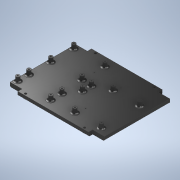
# Autodesk Inventor part: Base_Componentes_Arduino
Saved by Autodesk Inventor 2020 (Build 240168000, 168)
## iProperties
Created: 2021-06-24
Part Number: Base_Componentes_Arduino
Material: Plástico PC/ABS
Document SubType Name: Modeling
Designer: JCarlos
Density: 0.357273 g/cm^3
Appearance: Brilhosa - Preta
Author: JCarlos
Autodesk Inventor part; units mm, degrees
ref_plane "YZ Plane" through (0, 0, 0) normal (1, 0, 0) x (0, 1, 0)
ref_plane "XZ Plane" through (0, 0, 0) normal (0, 1, 0) x (-1, 0, 0)
ref_plane "XY Plane" through (0, 0, 0) normal (0, 0, 1) x (1, 0, 0)
sketch "Esboço1" plane through (0, 0, 0) normal (0, 1, 0) x (-1, 0, 0)
  line L0 (60, -62.5) -> (-60, -62.5)
  line L1 (-80, -55.5) -> (-80, 55.5)
  line L2 (-60, 62.5) -> (60, 62.5)
  line L3 (80, 55.5) -> (80, -55.5)
  line L4 (80, -55.5) -> (60, -55.5)
  line L5 (60, -55.5) -> (60, -62.5)
  line L6 (0, 0) -> (0, -37.6939)
  line L7 (0, 0) -> (28.8208, 0)
  line L8 (-80, -55.5) -> (-60, -55.5)
  line L9 (-60, -55.5) -> (-60, -62.5)
  line L10 (80, 55.5) -> (60, 55.5)
  line L11 (60, 55.5) -> (60, 62.5)
  line L12 (-60, 55.5) -> (-60, 62.5)
  line L13 (-80, 55.5) -> (-60, 55.5)
  point P0 (80, 0)
  point P1 (0, -62.5)
  point P2 (-80, 0)
  point P3 (80, 0)
  dimension "d2" = 7
  dimension "d4" = 20
  dimension "d5" = 125
  dimension "d6" = 111
  dimension "d7" = 160
  constraints: 28 end point, 9 symmetric about line, 4 midpoint, 3 horizontal, 3 horizontal alignment, 2 parallel, 2 perpendicular, 1 point on line, 1 vertical, 1 vertical alignment
  measures "d2" distance between parallel lines of L0 L4
  measures "d4" distance of L3.end L4.end
  measures "d5" distance between parallel lines of L2 L0
  measures "d6" distance of L3.start L3.end
  measures "d7" distance between parallel lines of L1 L3
extrude "Extrusão1" add sketch "Esboço1" along normal blind 6.5
sketch "Esboço3" plane through (0, 0, 0) normal (0, -1, 0) x (1, 0, 0)
  line L0 (-60, 62.5) -> (60, 62.5) projected
  line L1 (60, 62.5) -> (60, 55.5) projected
  point P0 (0, 0)
  point P1 (50, 59.25)
  dimension "d10" = 3.25
  dimension "d11" = 10
  measures "d10" distance from line of L0 point (50, 59.25)
  measures "d11" distance from line of L1 point (50, 59.25)
hole "Furo1" at (50, 0, 59.25) direction (0, 1, 0) diameter 3.5 end through all counterbore diameter 6 counterbore depth 2.5
mirror "Espelhamento1" about plane through (0, 0, 0) normal (1, 0, 0) of "Furo1"
mirror "Espelhamento2" about plane through (0, 0, 0) normal (0, 0, 1) of "Furo1", "Espelhamento1"
fillet "Arredondamento1" radius 2 4 edges at (-80, 0, 0) (0, 0, 62.5) (0, 0, -62.5) (80, 0, 0)
sketch "Esboço4" plane through (0, 6.5, 0) normal (0, 1, 0) x (1, 0, 0)
  circle A0 centre (20, 19.5) radius 3
  circle A1 centre (65, 19.5) radius 3
  circle A2 centre (20, -45.5) radius 3
  circle A3 centre (65, -45.5) radius 3
  line L0 (80, -55.5) -> (80, 55.5) projected
  circle A4 centre (-75, 47.5) radius 3
  circle A5 centre (-22, 47.5) radius 3
  circle A6 centre (-75, 8.5) radius 3
  circle A7 centre (-22, 8.5) radius 3
  line L1 (-80, 55.5) -> (-80, -55.5) projected
  line L2 (-60, 55.5) -> (-80, 55.5) projected
  line L3 (-80, -55.5) -> (-60, -55.5) projected
  circle A8 centre (-75, -28.5) radius 3
  circle A9 centre (-75, -47.5) radius 3
  circle A10 centre (-19, -28.5) radius 3
  circle A11 centre (-19, -47.5) radius 3
  circle A12 centre (-5, 7.5) radius 3
  circle A13 centre (-5, -7.5) radius 3
  line L4 (60, -55.5) -> (80, -55.5) projected
  point P0 (0, 0)
  dimension "d21" = 65
  dimension "d22" = 6
  dimension "d24" = 15
  dimension "d25" = 53
  dimension "d26" = 39
  dimension "d27" = 5
  dimension "d28" = 8
  dimension "d30" = 19
  dimension "d31" = 8
  dimension "d32" = 56
  dimension "d35" = 15
  dimension "d36" = 7.5
  dimension "d39" = 5
  dimension "d69" = 45
  dimension "d71" = 10
  constraints: 14 centre point, 13 equal radius, 8 vertical alignment, 6 horizontal alignment
  measures "d21" distance of A2.centre A0.centre
  measures "d22" diameter of A0
  measures "d24" distance from line of L0 A1.centre
  measures "d25" distance of A5.centre A4.centre
  measures "d26" distance of A6.centre A4.centre
  measures "d27" distance from line of L1 A4.centre
  measures "d28" distance from line of L2 A4.centre
  measures "d30" distance of A9.centre A8.centre
  measures "d31" distance from line of L3 A9.centre
  measures "d32" distance of A10.centre A8.centre
  measures "d35" distance of A13.centre A12.centre
  measures "d36" vertical distance of point (0, 0) A12.centre
  measures "d39" horizontal distance of point (0, 0) A12.centre
  measures "d69" distance of A1.centre A0.centre
  measures "d71" distance from line of L4 A3.centre
extrude "Extrusão2" add sketch "Esboço4" along normal blind 8
fillet "Arredondamento2" radius 3 14 edges at (-78, 6.5, -47.5) (-25, 6.5, -47.5) (-78, 6.5, -8.5) (-78, 6.5, 28.5) (-78, 6.5, 47.5) (-25, 6.5, -8.5) (-22, 6.5, 28.5) (-22, 6.5, 47.5) (17, 6.5, 45.5) (-8, 6.5, 7.5) (-8, 6.5, -7.5) (17, 6.5, -19.5) (62, 6.5, -19.5) (62, 6.5, 45.5)
sketch "Esboço5" plane through (0, 0, 0) normal (0, -1, 0) x (1, 0, 0)
  circle A0 centre (-22.5, 30) radius 0.75
  circle A1 centre (22.5, 30) radius 0.75
  line L0 (0, 0) -> (-9.3939, 0)
  circle A2 centre (-22.5, -30) radius 0.75
  circle A3 centre (22.5, -30) radius 0.75
  dimension "d40" = 1.5
  dimension "d41" = 45
  dimension "d42" = 60
  dimension "d43" = 22.5
  constraints: 4 centre point, 2 end point, 2 symmetric about line, 1 equal radius, 1 horizontal, 1 horizontal alignment, 2 other
  measures "d40" diameter of A0
  measures "d41" distance of A1.centre A0.centre
  measures "d42" diameter of A0.centre L0
  measures "d43" horizontal distance of L0.start A0.centre
extrude "Extrusão3" cut sketch "Esboço5" against normal through all
sketch "Esboço6" plane through (-75, 14.5, -47.5) normal (0, 1, 0) x (1, 0, 0)
  circle A0 centre (0, 0) radius 3 projected
  point P0 (75, -47.5)
  constraints: 1 coincident
hole "Furo2" at (-75, 14.5, -47.5) direction (0, -1, 0) diameter 2.25 depth 8 tip angle 118
sketch "Esboço7" plane through (-22, 14.5, -47.5) normal (0, 1, 0) x (1, 0, 0)
  circle A0 centre (0, 0) radius 3 projected
  point P0 (22, -47.5)
  constraints: 1 coincident
hole "Furo3" at (-22, 14.5, -47.5) direction (0, -1, 0) diameter 2.25 depth 8 tip angle 118
sketch "Esboço8" plane through (-75, 14.5, -8.5) normal (0, 1, 0) x (1, 0, 0)
  circle A0 centre (0, 0) radius 3 projected
  circle A1 centre (0, -37) radius 3 projected
  circle A2 centre (0, -56) radius 3 projected
  circle A3 centre (56, -56) radius 3 projected
  circle A4 centre (56, -37) radius 3 projected
  circle A5 centre (53, 0) radius 3 projected
  circle A6 centre (70, -16) radius 3 projected
  circle A7 centre (70, -1) radius 3 projected
  circle A8 centre (95, -54) radius 3 projected
  circle A9 centre (140, -54) radius 3 projected
  circle A10 centre (140, 11) radius 3 projected
  circle A11 centre (95, 11) radius 3 projected
  point P0 (75, -8.5)
  constraints: 12 coincident
hole "Furo4" at (-75, 14.5, -8.5) at (-75, 14.5, 28.5) at (-75, 14.5, 47.5) at (-19, 14.5, 47.5) at (-19, 14.5, 28.5) at (-22, 14.5, -8.5) at (-5, 14.5, 7.5) at (-5, 14.5, -7.5) at (20, 14.5, 45.5) at (65, 14.5, 45.5) at (65, 14.5, -19.5) at (20, 14.5, -19.5) direction (0, -1, 0) diameter 2.25 depth 8 tip angle 118
equation "\"d36\" = 0.5 * d35"
equation "\"d43\" = 0.5 * d41"
